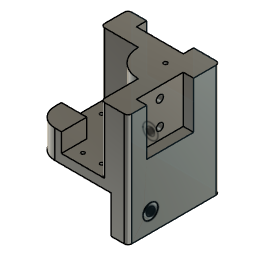
idler-profile connector 1 (Autodesk Fusion 360 design; units mm, degrees)
Autodesk Fusion 360 part; units mm, degrees
note: some values were not read from the file. Set by a fixed rule: which sketch regions a step uses.
sketch "Sketch1" plane through (0, 0, 0) normal (0, 0, 1) x (1, 0, 0)
  line L0 (20, -20) -> (-10, -20)
  line L1 (-20, -10) -> (-20, 20)
  line L2 (-20, 20) -> (20, 20)
  line L3 (20, 20) -> (20, -20)
  line L4 (20, -20) -> (-20, 20) construction
  line L5 (-20, -20) -> (20, 20) construction
  circle A0 centre (14.5, 14.5) radius 1.5
  line L6 (14.5, -20) -> (14.5, -20)
  line L7 (14.5, -20) -> (14.5, 14.5)
  line L8 (14.5, 14.5) -> (14.5, 14.5)
  line L9 (14.5, 14.5) -> (14.5, -20)
  line L10 (-6.5, -20) -> (-6.5, -6.5)
  line L11 (-6.5, -6.5) -> (-20, -6.5)
  line L12 (14.5, 14.5) -> (-20, 14.5)
  arc A1 (-20, -10) -> (-10, -20) centre (-10, -10) ccw
  line L13 (0, 14.5) -> (0, 0)
  line L14 (14.5, 0) -> (0, 0)
  circle A2 centre (14.5, 14.5) radius 7
  circle A3 centre (14.5, 14.5) radius 14.5
  line L15 (29, 29) -> (29, -20)
  line L16 (29, -20) -> (20, -20)
  line L17 (29, 29) -> (-20, 29)
  line L18 (-20, 29) -> (-20, 20)
  line L19 (21.5, 21.5) -> (21.5, -20)
  line L20 (21.5, 21.5) -> (-20, 21.5)
  line L21 (14.5, 0) -> (20, 0)
  line L22 (0, 14.5) -> (0, 20)
  circle A4 centre (-1, -14) radius 0.9
  circle A5 centre (9, -14) radius 0.9
  circle A6 centre (-14, -1) radius 0.9
  circle A7 centre (-14, 9) radius 0.9
  dimension "d1" = 5.5
  dimension "d3" = 40
  dimension "d8" = 3
  dimension "d12" = 10
  dimension "d37" = 14
  dimension "d72" = 1.8
  dimension "d73" = 1.8
  constraint horizontal L0
  constraint perpendicular L0 L1
  constraint parallel L0 L2
  constraint parallel L1 L3
  constraint coincident L4 L13.end
  constraint coincident L5 L13.end
  constraint coincident L13.end L14.end
  constraint coincident L5 A0.centre
  constraint vertical L7
  constraint vertical L9
  constraint coincident A0.centre L7.end
  constraint coincident L0 L6.start
  constraint coincident L0 L10.start
  constraint coincident L5 L10.end
  constraint perpendicular L0 L10
  constraint coincident L1 L11.end
  constraint perpendicular L1 L11
  constraint coincident L1 L12.end
  constraint coincident L5.start L1
  constraint coincident L5.start L0
  constraint tangent L1 A1
  constraint tangent L0 A1
  constraint coincident L12 L13.start
  constraint coincident L9 L14.start
  constraint horizontal L14
  constraint concentric A0 A2
  constraint concentric A0 A3
  constraint coincident L13.start A3
  constraint perpendicular L7 L12
  constraint perpendicular L0 L15
  constraint parallel L0 L16
  constraint perpendicular L15 L17
  constraint coincident L16 L19.end
  constraint perpendicular L16 L19
  constraint coincident L18 L20.end
  constraint perpendicular L18 L20
  constraint midpoint L3 L21.end
  constraint parallel L14 L21
  constraint midpoint L2 L22.end
  constraint tangent A3 L22
  constraint symmetric L5 A4 A6
  constraint symmetric L5 A5 A7
  measures "d1" distance of L2 A0.centre
  measures "d3" distance of L0.start L5.start
  measures "d8" diameter of A0
  measures "d12" radius of A1
  measures "d37" diameter of A2
  measures "d72" diameter of A5
  measures "d73" diameter of A4
extrude "Extrude1" add sketch "Sketch1" against normal blind 20 contours L3 A3 L16 L19 | L3 A3 L21 | A3 L15 L16 L19 | L7 L9 L12 A2 A3 | L13 L14 A3 | L3 L7 L9 A2 A3 | L3 A2 A3 L19 | A3 L19 L20 | A0 L7 L9 L12 A2 | L2 L3 A0 L7 L9 L12 A2 | L2 L12 A2 A3 | L2 A3 L22 | L3 A2 | A3 L15 L17 | L2 L3 A2 L19 L20 | A0 L7 L9 L12 | A0 L7 L9 L12 | L2 A2 A3 L20 | L2 A3 L18 L20 | L2 L3 A2 | A3 L17 L18 L20 | L2 A2
extrude "Extrude2" add sketch "Sketch1" along normal blind 5
extrude "Extrude3" add sketch "Sketch1" along normal blind 35 from surface at 5 contours L0 L3 L7 L9 L21 | L3 A3 L16 L19 | L3 A3 L21 | A3 L15 L16 L19 | L7 L9 L12 A2 A3 | L3 L7 L9 A2 A3 | L3 A2 A3 L19 | A3 L19 L20 | A0 L7 L9 L12 A2 | L2 L3 A0 L7 L9 L12 A2 | L2 L12 A2 A3 | L2 A3 L22 | L1 L2 L12 L22 | L3 A2 | A3 L15 L17 | L2 L3 A2 L19 L20 | L2 A2 A3 L20 | L2 A3 L18 L20 | L2 L3 A2 | A3 L17 L18 L20 | L2 A2
extrude "Extrude4" add sketch "Sketch1" along normal blind 10 from surface at 5 contours L0 L1 L10 L11 A1
sketch "Sketch2" plane through (0, 0, 40) normal (0, 0, 1) x (-1, 0, 0)
  line L0 (20, -14.5) -> (0, -14.5)
  arc A0 (0, -14.5) -> (-14.5, 0) centre (-14.5, -14.5) ccw
  circle A1 centre (-14.5, -14.5) radius 1.5
  line L1 (-14.5, 20) -> (-29, 20)
  line L2 (-29, 20) -> (-29, -29)
  line L3 (-29, -29) -> (20, -29)
  line L4 (20, -29) -> (20, -20)
  line L5 (20, -20) -> (20, -14.5)
  line L6 (-14.5, 0) -> (-14.5, 20)
  line L7 (10, -29) -> (-15, -29)
  line L8 (-15, -29) -> (-15, -23.5)
  line L9 (-15, -23.5) -> (10, -23.5)
  line L10 (10, -23.5) -> (10, -29)
  line L11 (-29, 10) -> (-23.5, 10)
  line L12 (-23.5, 10) -> (-23.5, -15)
  line L13 (-23.5, -15) -> (-29, -15)
  line L14 (-29, -15) -> (-29, 10)
  dimension "d39" = 9
  dimension "d40" = 9
  constraint horizontal L7
  constraint vertical L8
  constraint horizontal L9
  constraint vertical L10
  constraint coincident L3 L7.start
  constraint horizontal L11
  constraint vertical L12
  constraint horizontal L13
  constraint vertical L14
  constraint coincident L2 L11.start
  measures "d39" distance of A0.centre L12
  measures "d40" distance of A0.centre L9
extrude "Extrude5" cut sketch "Sketch2" against normal blind 25 contours L3 L7 L8 L9 L10 | L2 L11 L12 L13 L14
sketch "Sketch5" plane through (23.5, 0, 0) normal (1, 0, 0) x (0, 1, 0)
  line L0 (15, 40) -> (-10, 40)
  line L1 (-10, 40) -> (-10, 15)
  line L2 (-10, 15) -> (15, 15)
  line L3 (15, 15) -> (15, 40)
  circle A0 centre (2.5, 21) radius 1.9
  circle A1 centre (2.5, 34) radius 1.9
  dimension "d41" = 6
  dimension "d42" = 6
  dimension "d43" = 3.8
  dimension "d44" = 3.8
  measures "d41" distance of L0 A1.centre
  measures "d42" distance of L2 A0.centre
  measures "d43" diameter of A1
  measures "d44" diameter of A0
extrude "Extrude8" cut sketch "Sketch5" against normal blind 5 contours A0 | A1
sketch "Sketch6" plane through (0, 23.5, 0) normal (0, 1, 0) x (-1, 0, 0)
  line L0 (10, 40) -> (-15, 40)
  line L1 (-15, 40) -> (-15, 15)
  line L2 (-15, 15) -> (10, 15)
  line L3 (10, 15) -> (10, 40)
  circle A0 centre (-2.5, 34) radius 1.9
  circle A1 centre (-2.5, 21) radius 1.9
  dimension "d47" = 6
  dimension "d48" = 6
  dimension "d49" = 3.8
  dimension "d50" = 3.8
  measures "d47" distance of L2 A1.centre
  measures "d48" distance of L0 A0.centre
  measures "d49" diameter of A0
  measures "d50" diameter of A1
extrude "Extrude9" cut sketch "Sketch6" against normal blind 5 contours A0 | A1
fillet "Fillet1" radius 2 5 edges at (29, 29, 10) (-20, 29, 10) (-20, 14.5, 22.5) (14.5, -20, 22.5) (29, -20, 10)
sketch "Sketch7" plane through (29, 0, 0) normal (1, 0, 0) x (0, 1, 0)
  line L0 (-18, 40) -> (-18, -20)
  line L1 (-18, -20) -> (27, -20)
  line L2 (27, -20) -> (27, 40)
  line L3 (27, 40) -> (15, 40)
  line L4 (15, 40) -> (15, 15)
  line L5 (15, 15) -> (-10, 15)
  line L6 (-10, 15) -> (-10, 40)
  line L7 (-10, 40) -> (-18, 40)
  circle A0 centre (-8, -10) radius 2.1
  circle A1 centre (-8, -10) radius 4
  dimension "d55" = 4.2
  dimension "d56" = 8
  dimension "d57" = 10
  dimension "d58" = 10
  constraint concentric A0 A1
  measures "d55" diameter of A0
  measures "d56" diameter of A1
  measures "d57" distance of L1 A0.centre
  measures "d58" distance of L0 A0.centre
extrude "Extrude10" cut sketch "Sketch7" against normal blind 14.5 contours A0
extrude "Extrude11" cut sketch "Sketch7" against normal blind 5 contours A1
sketch "Sketch8" plane through (0, 29, 0) normal (0, 1, 0) x (-1, 0, 0)
  line L0 (18, -20) -> (18, 40)
  line L1 (18, 40) -> (10, 40)
  line L2 (10, 40) -> (10, 15)
  line L3 (10, 15) -> (-15, 15)
  line L4 (-15, 15) -> (-15, 40)
  line L5 (-15, 40) -> (-27, 40)
  line L6 (-27, 40) -> (-27, -20)
  line L7 (-27, -20) -> (18, -20)
  circle A0 centre (8, -10) radius 2.1
  circle A1 centre (8, -10) radius 4
  dimension "d63" = 4.2
  dimension "d64" = 8
  dimension "d65" = 10
  dimension "d66" = 10
  constraint concentric A0 A1
  measures "d63" diameter of A0
  measures "d64" diameter of A1
  measures "d65" distance of L7 A0.centre
  measures "d66" distance of L0 A0.centre
extrude "Extrude12" cut sketch "Sketch8" against normal blind 14.5 contours A0
extrude "Extrude13" cut sketch "Sketch8" against normal blind 5 contours A1
move_face "OffsetFaces1" offset 0.5 1 faces at (15.9981, 14.5748, 16.6667)
